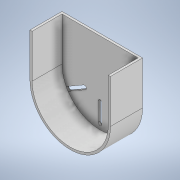
# Autodesk Inventor part: TapaEje
Saved by Autodesk Inventor 2020 (Build 240168000, 168)
## iProperties
Created: 2019-11-12
Part Number: TapaEje
Material: Genérico
Document SubType Name: Modeling
Designer: Usuario
Density: 1 g/cm^3
Appearance: Valor por defecto
Author: Usuario
## iProperties of the stored document _3DPrint.ipt
Created: 2019-11-12
Part Number: _3DPrint
Material: Genérico
Document SubType Name: Modeling
Designer: Usuario
Density: 1 g/cm^3
Appearance: Valor por defecto
Author: Usuario
Autodesk Inventor part; units mm, degrees
ref_plane "YZ Plane" through (0, 0, 0) normal (1, 0, 0) x (0, 1, 0)
ref_plane "XZ Plane" through (0, 0, 0) normal (0, 1, 0) x (-1, 0, 0)
ref_plane "XY Plane" through (0, 0, 0) normal (0, 0, 1) x (1, 0, 0)
sketch "Boceto1" plane through (0, 0, 0) normal (0, 0, 1) x (1, 0, 0)
  arc A0 (-54, 0) -> (54, 0) centre (0, 0) ccw
  line L0 (-54, 0) -> (-54, 58)
  line L1 (54, 58) -> (54, 0)
  arc A1 (54, 0) -> (-54, 0) centre (0, 0) ccw construction
  line L2 (0, -54) -> (0, 58) construction
  line L3 (54, 58) -> (-54, 58)
  line L4 (54, 58) -> (54, 58)
  line L5 (-54, 58) -> (-54, 58)
  line L6 (-54, 58) -> (0, 58) construction
  line L7 (0, 58) -> (54, 58) construction
  line L8 (0, -43.4382) -> (0, -18.4382) construction
  line L9 (2.5, -43.4382) -> (2.5, -18.4382)
  line L10 (-2.5, -18.4382) -> (-2.5, -43.4382)
  arc A2 (-2.5, -43.4382) -> (2.5, -43.4382) centre (0, -43.4382) ccw
  arc A3 (2.5, -18.4382) -> (-2.5, -18.4382) centre (0, -18.4382) ccw
  line L11 (0, 0) -> (-46.7654, -27) construction
  line L12 (0, 0) -> (46.7654, -27) construction
  line L13 (-42.4352, -24.5) -> (-20.7846, -12) construction
  line L14 (-41.1852, -26.6651) -> (-19.5346, -14.1651)
  line L15 (-22.0346, -9.8349) -> (-43.6852, -22.3349)
  arc A4 (-43.6852, -22.3349) -> (-41.1852, -26.6651) centre (-42.4352, -24.5) ccw
  arc A5 (-19.5346, -14.1651) -> (-22.0346, -9.8349) centre (-20.7846, -12) ccw
  line L16 (42.4352, -24.5) -> (20.7846, -12) construction
  line L17 (43.6852, -22.3349) -> (22.0346, -9.8349)
  line L18 (19.5346, -14.1651) -> (41.1852, -26.6651)
  arc A6 (41.1852, -26.6651) -> (43.6852, -22.3349) centre (42.4352, -24.5) ccw
  arc A7 (22.0346, -9.8349) -> (19.5346, -14.1651) centre (20.7846, -12) ccw
  point P0 (0, -30.9382)
  point P1 (-31.6099, -18.25)
  point P2 (31.6099, -18.25)
  dimension "d0" = 108
  dimension "d2" = 112
  dimension "d11" = 60
  dimension "d12" = 60
  dimension "d13" = 5
  dimension "d14" = 5
  dimension "d15" = 5
  dimension "d16" = 25
  dimension "d17" = 25
  dimension "d18" = 25
  dimension "d19" = 5
  dimension "d20" = 5
  constraints: 44 end point, 19 point on circle, 14 tangent, 8 centre point, 7 point on line, 4 midpoint, 4 parallel, 4 perpendicular, 2 vertical, 1 coincident, 1 collinear
  measures "d0" diameter of A0
  measures "d2" distance of L2.end L2.start
  measures "d11" angle of L12 L2
  measures "d12" angle of L2 L11
  measures "d13" distance between parallel lines of L9 L10
  measures "d14" distance between parallel lines of L17 L18
  measures "d15" distance between parallel lines of L14 L15
  measures "d16" distance of L8.end L8.start
  measures "d17" distance of L17.start L17.end
  measures "d18" distance of L15.start L15.end
  measures "d19" distance of L11.end L13.start
  measures "d20" distance of L12.end L16.start
extrude "Extrusión2" add sketch "Boceto1" along normal blind 3
sketch "Boceto2" plane through (0, 0, 3) normal (0, 0, 1) x (1, 0, 0)
  arc A0 (-54, 0) -> (54, 0) centre (0, 0) ccw projected
  line L0 (54, 0) -> (54, 58) projected
  line L1 (54, 58) -> (-54, 58) construction
  line L2 (-54, 58) -> (-54, 0) projected
  arc A1 (-51, 0) -> (51, 0) centre (0, 0) ccw
  line L3 (51, 0) -> (51, 55)
  line L4 (51, 55) -> (-51, 55) construction
  line L5 (-51, 55) -> (-51, 0)
  line L6 (-51, 55) -> (-51, 58)
  line L7 (51, 55) -> (51, 58)
  line L8 (54, 58) -> (51, 58)
  line L9 (54, 58) -> (-54, 58) projected
  line L10 (-51, 58) -> (-54, 58)
  dimension "d8" = 3
  constraints: 14 end point, 2 point on circle, 2 point on line, 2 vertical, 1 centre point, 1 collinear, 1 horizontal, 3 other
  measures "d8" distance between parallel lines of L2 L5
extrude "Extrusión3" add sketch "Boceto2" along normal blind 40 contours L2 L9 L6 L5 A1 L3 L7 L8 L0 A0
sketch "Boceto3" plane through (0, 0, 0) normal (0, 0, -1) x (-1, 0, 0)
  circle A0 centre (0, 0) radius 12.5
  dimension "d21" = 25
  constraints: 1 centre point, 1 coincident
  measures "d21" diameter of A0
extrude "Extrusión4" add sketch "Boceto3" along normal blind 10 draft -20
fillet "Empalme1" radius 2 1 edges at (8.8603, 0, -10)
